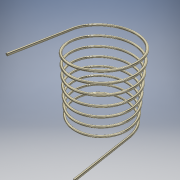
# Autodesk Inventor part: Coil
Saved by Autodesk Inventor 2017 (Build 210142000, 142)
## iProperties
Created: 2016-12-16
Part Number: Coil
Material: Generic
Document SubType Name: Modeling
Designer: ge937963
Density: 1 g/cm^3
Appearance: Nickel
Author: ge937963
Autodesk Inventor part; units mm, degrees
ref_plane "YZ Plane" through (0, 0, 0) normal (1, 0, 0) x (0, 1, 0)
ref_plane "XZ Plane" through (0, 0, 0) normal (0, 1, 0) x (-1, 0, 0)
ref_plane "XY Plane" through (0, 0, 0) normal (0, 0, 1) x (1, 0, 0)
sketch "Sketch1" plane through (0, 0, 0) normal (0, 0, 1) x (1, 0, 0)
  circle A0 centre (3.302, 0) radius 0.127
  line L0 (3.175, 0) -> (3.175, -0.1101)
  point P0 (0, 0)
  dimension "d0" = 0.254
  dimension "d1" = 3.175
  constraints: 2 end point, 1 horizontal alignment, 1 vertical, 2 other
  measures "d1" distance from line of point (0, 0) L0
coil "Coil1" sketch "Sketch1" operation add axis through (0, -10, 0) along (0, 1, 0) pitch 1.016 turns 7.5 hand right
sketch "Sketch2" plane through (-3.302, 7.62, 0) normal (0, 0, 1) x (1, 0, 0)
  circle A0 centre (0, 0) radius 0.127
  circle A1 centre (6.604, -7.62) radius 0.127 projected
  circle A2 centre (6.604, -7.62) radius 0.127
  point P0 (3.302, -7.62)
  point P1 (6.731, -7.62)
  point P2 (-0.127, 0)
  constraints: 2 centre point, 1 coincident, 1 horizontal alignment, 2 other
extrude "Extrusion1" add sketch "Sketch2" along normal blind 6.35
body "Solid1"
